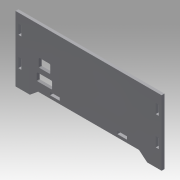
# Autodesk Inventor part: back_instrumentboard
Saved by Autodesk Inventor 2019.3 (Build 233278000, 278)
## iProperties
Created: 2019-05-28
Part Number: back_instrumentboard
Material: Generic
Document SubType Name: Modeling
Designer: Dave
Density: 1 g/cm^3
Appearance: Default
Author: Dave
Autodesk Inventor part; units mm, degrees
ref_plane "YZ Plane" through (0, 0, 0) normal (1, 0, 0) x (0, 1, 0)
ref_plane "XZ Plane" through (0, 0, 0) normal (0, 1, 0) x (-1, 0, 0)
ref_plane "XY Plane" through (0, 0, 0) normal (0, 0, 1) x (1, 0, 0)
sketch "Sketch1" plane through (0, 0, 0) normal (0, 0, 1) x (1, 0, 0)
  line L0 (0, 0) -> (152, 0)
  line L1 (152, 0) -> (152, 68)
  line L2 (152, 68) -> (0, 68)
  line L3 (0, 68) -> (0, 0)
  line L4 (36, 13) -> (46, 13)
  line L5 (46, 13) -> (46, 10)
  line L6 (46, 10) -> (36, 10)
  line L7 (36, 10) -> (36, 13)
  line L8 (106, 13) -> (116, 13)
  line L9 (116, 13) -> (116, 10)
  line L10 (116, 10) -> (106, 10)
  line L11 (106, 10) -> (106, 13)
  line L12 (3, 28) -> (6.1, 28)
  line L13 (6.1, 28) -> (6.1, 18)
  line L14 (6.1, 18) -> (3, 18)
  line L15 (3, 18) -> (3, 28)
  line L16 (3, 58) -> (6.1, 58)
  line L17 (6.1, 58) -> (6.1, 48)
  line L18 (6.1, 48) -> (3, 48)
  line L19 (3, 48) -> (3, 58)
  line L20 (145.9, 58) -> (149, 58)
  line L21 (149, 58) -> (149, 48)
  line L22 (149, 48) -> (145.9, 48)
  line L23 (145.9, 48) -> (145.9, 58)
  line L24 (145.9, 28) -> (149, 28)
  line L25 (149, 28) -> (149, 18)
  line L26 (149, 18) -> (145.9, 18)
  line L27 (145.9, 18) -> (145.9, 28)
  line L28 (23.5, 7) -> (128.5, 7)
  line L29 (128.5, 7) -> (137, 0)
  line L30 (23.5, 7) -> (15, 0)
  dimension "d0" = 3
  dimension "d1" = 10
  dimension "d2" = 60
  dimension "d3" = 10
  dimension "d4" = 152
  dimension "d5" = 36
  dimension "d6" = 36
  dimension "d7" = 3.1
  dimension "d8" = 10
  dimension "d9" = 20
  dimension "d10" = 5
  dimension "d11" = 10
  dimension "d12" = 3
  dimension "d13" = 3
  dimension "d14" = 3
  dimension "d15" = 15
  dimension "d16" = 15
  dimension "d17" = 105
  constraints: 62 end point, 14 parallel, 8 horizontal, 8 point on line, 7 perpendicular, 6 equal length, 2 collinear
  measures "d0" distance of L6.end L4.start
  measures "d1" distance of L4.start L4.end
  measures "d2" distance between parallel lines of L11 L5
  measures "d3" distance between parallel lines of L0 L6
  measures "d4" distance between parallel lines of L1 L3
  measures "d5" distance between parallel lines of L1 L9
  measures "d6" distance between parallel lines of L3 L7
  measures "d7" distance of L16.start L16.end
  measures "d8" distance of L16.end L17.end
  measures "d9" distance between parallel lines of L12 L18
  measures "d10" distance between parallel lines of L4 L14
  measures "d11" distance between parallel lines of L2 L16
  measures "d12" distance between parallel lines of L1 L21
  measures "d13" distance between parallel lines of L3 L19
  measures "d14" distance between parallel lines of L28 L6
  measures "d15" distance from line of L3 L30.end
  measures "d16" distance from line of L1 L29.end
  measures "d17" distance of L28.start L28.end
extrude "Extrusion1" add sketch "Sketch1" along normal blind 3 contours L3 L2 L1 L0 L29 L28 L30
sketch "Sketch2" plane through (0, 0, 3) normal (0, 0, 1) x (1, 0, 0)
  line L0 (25.19, 38.1) -> (35.19, 38.1)
  line L1 (36.19, 37.1) -> (36.19, 30.1)
  line L2 (35.19, 29.1) -> (25.19, 29.1)
  line L3 (24.19, 30.1) -> (24.19, 37.1)
  line L4 (6.1, 28) -> (6.1, 18) projected
  line L5 (36, 13) -> (46, 13) projected
  line L6 (23.5, 7) -> (128.5, 7) projected
  arc A0 (25.19, 38.1) -> (24.19, 37.1) centre (25.19, 37.1) ccw
  arc A1 (36.19, 37.1) -> (35.19, 38.1) centre (35.19, 37.1) ccw
  arc A2 (35.19, 29.1) -> (36.19, 30.1) centre (35.19, 30.1) ccw
  arc A3 (24.19, 30.1) -> (25.19, 29.1) centre (25.19, 30.1) ccw
  line L7 (16.85, 23) -> (43.35, 23)
  line L8 (43.35, 23) -> (43.35, 12)
  line L9 (43.35, 12) -> (16.85, 12)
  line L10 (16.85, 12) -> (16.85, 23)
  line L11 (3, 28) -> (6.1, 28) projected
  line L12 (23.1, 24) -> (37.1, 24)
  line L13 (38.1, 23) -> (38.1, 17)
  line L14 (37.1, 16) -> (23.1, 16)
  line L15 (22.1, 17) -> (22.1, 23)
  arc A4 (23.1, 24) -> (22.1, 23) centre (23.1, 23) ccw
  arc A5 (22.1, 17) -> (23.1, 16) centre (23.1, 17) ccw
  arc A6 (37.1, 16) -> (38.1, 17) centre (37.1, 17) ccw
  arc A7 (38.1, 23) -> (37.1, 24) centre (37.1, 23) ccw
  point P0 (0, 0)
  point P1 (24.19, 38.1)
  point P2 (36.19, 29.1)
  point P3 (36.19, 38.1)
  point P4 (24.19, 29.1)
  point P5 (30.19, 38.1)
  point P6 (24.19, 33.6)
  point P7 (22.1, 24)
  point P8 (38.1, 16)
  point P9 (38.1, 24)
  point P10 (22.1, 16)
  point P11 (30.1, 23)
  point P12 (30.1, 24)
  dimension "d20" = 24.09
  dimension "d23" = 12
  dimension "d24" = 9
  dimension "d28" = 20.6
  dimension "d29" = 1
  dimension "d30" = 10.75
  dimension "d31" = 37.25
  dimension "d32" = 5
  dimension "d33" = 5
  dimension "d34" = 16
  dimension "d35" = 3
  dimension "d36" = 8
  dimension "d37" = 1
  constraints: 24 end point, 16 point on circle, 16 point on line, 16 tangent, 8 centre point, 6 equal radius, 6 parallel, 4 midpoint, 3 horizontal, 3 perpendicular, 1 vertical alignment
  measures "d20" distance from line of L4 point (30.19, 38.1)
  measures "d23" distance of point (24.19, 38.1) point (36.19, 38.1)
  measures "d24" distance of point (36.19, 38.1) point (36.19, 29.1)
  measures "d28" distance from line of L5 point (24.19, 33.6)
  measures "d29" radius of A0
  measures "d30" distance between parallel lines of L10 L4
  measures "d31" distance between parallel lines of L4 L8
  measures "d32" distance between parallel lines of L6 L9
  measures "d33" distance between parallel lines of L11 L7
  measures "d34" distance of point (22.1, 24) point (38.1, 24)
  measures "d35" distance between parallel lines of L5 L14
  measures "d36" distance of point (38.1, 24) point (38.1, 16)
  measures "d37" radius of A4
extrude "Extrusion2" cut sketch "Sketch2" against normal blind 10 contours L0 A1 L1 A2 L2 A3 L3 A0 | A4 L12 A7 L7 | L7 L13 A6 L14 A5 L15
body "Solid1"
